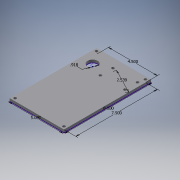
# Autodesk Inventor part: eboardpartisland
Saved by Autodesk Inventor 2016 (Build 200138000, 138)
## iProperties
Created: 2016-01-21
Part Number: eboardpartisland
Material: Generic
Document SubType Name: Modeling
Designer: Administrator
Density: 1 g/cm^3
Appearance: Default
Author: Administrator
Autodesk Inventor part; units mm, degrees
ref_plane "YZ Plane" through (0, 0, 0) normal (1, 0, 0) x (0, 1, 0)
ref_plane "XZ Plane" through (0, 0, 0) normal (0, 1, 0) x (-1, 0, 0)
ref_plane "XY Plane" through (0, 0, 0) normal (0, 0, 1) x (1, 0, 0)
sketch "Sketch1" plane through (0, 0, 0) normal (0, 1, 0) x (-1, 0, 0)
  line L0 (63.5, -101.6) -> (-63.5, -101.6)
  line L1 (-63.5, -101.6) -> (-63.5, 101.6)
  line L2 (-63.5, 101.6) -> (63.5, 101.6)
  line L3 (63.5, 101.6) -> (63.5, -101.6)
  line L4 (63.5, -101.6) -> (-63.5, 101.6) construction
  line L5 (-63.5, -101.6) -> (63.5, 101.6) construction
  circle A0 centre (36.3684, -65.2364) radius 11.6586
  line L6 (57.15, 95.25) -> (-57.15, 95.25)
  line L7 (-57.15, 95.25) -> (-57.15, -95.25)
  line L8 (-57.15, -95.25) -> (57.15, -95.25)
  line L9 (57.15, -95.25) -> (57.15, 95.25)
  line L10 (57.15, 95.25) -> (-57.15, -95.25) construction
  line L11 (-57.15, 95.25) -> (57.15, -95.25) construction
  line L12 (2.7998, -50.5044) -> (-53.7731, -50.5044)
  line L13 (-53.7731, -50.5044) -> (-53.7731, -79.5676)
  line L14 (-53.7731, -79.5676) -> (2.7998, -79.5676)
  line L15 (2.7998, -79.5676) -> (2.7998, -50.5044)
  line L16 (2.7998, -79.5676) -> (-53.7731, -50.5044)
  point P0 (0, 0)
  point P1 (-25.0965, -65.2364)
  point P2 (-25.0965, -65.2364)
  dimension "d0" = 127
  dimension "d1" = 203.2
  dimension "d4" = 23.3172
  dimension "d7" = 114.3
  dimension "d8" = 190.5
  dimension "d18" = 63.6016
  constraints: 34 end point, 8 coincident, 6 parallel, 4 horizontal, 4 midpoint, 3 perpendicular, 1 centre point, 3 other
  measures "d0" distance of L1.end L2.end
  measures "d1" distance of L0.end L1.end
  measures "d4" diameter of A0
  measures "d7" distance of L8.end L7.end
  measures "d8" distance of L7.end L6.end
  measures "d18" distance of L16.start L16.end
extrude "Extrusion2" add sketch "Sketch1" along normal blind 6.35 contours L0 L1 L2 L3 | L9 L8 L7 L6 | L15 L16 L12 | L16 L14 L13
hole "Hole1" at (57.15, 0, -95.25) at (-57.15, 0, -95.25) at (-57.15, 0, 95.25) at (57.15, 0, 95.25) at (-2.7998, 0, -79.5676) at (-2.7998, 0, -50.5044) at (53.7731, 0, -50.5044) at (53.7731, 0, -79.5676) direction (0, 1, 0) diameter 6.35 end through all
body "Solid2"
